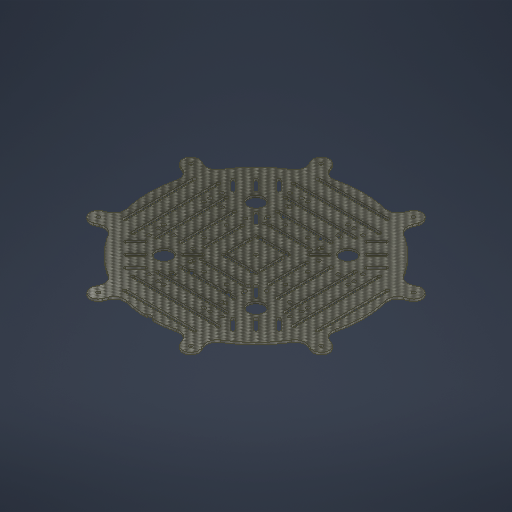
# Autodesk Inventor part: Body_Center_Plate
Saved by Autodesk Inventor 2025 (Build 290162010, 162A)
## iProperties
Created: 2023-12-04
Part Number: Body_Center_Plate
Material: GFRC
Document SubType Name: Modeling
Designer: dzw04
Density: 1.7 g/cm^3
Appearance: Carbon Fiber 1
Mass: 94.6856 g
Surface Area: 657.949 cm^2
Volume: 55.6974 cm^3
Author: dzw04
Autodesk Inventor part; units mm, degrees
ref_plane "YZ Plane" through (0, 0, 0) normal (1, 0, 0) x (0, 1, 0)
ref_plane "XZ Plane" through (0, 0, 0) normal (0, 1, 0) x (-1, 0, 0)
ref_plane "XY Plane" through (0, 0, 0) normal (0, 0, 1) x (1, 0, 0)
sketch "Sketch1" plane through (0, 0, 0) normal (0, 1, 0) x (-1, 0, 0)
  circle A0 centre (165, 165) radius 1.6
  circle A1 centre (121.9481, 268.9364) radius 1.6
  circle A2 centre (61.0636, 208.0519) radius 1.6
  circle A3 centre (61.0636, 121.9481) radius 1.6
  circle A4 centre (121.9481, 61.0636) radius 1.6
  circle A5 centre (208.0519, 61.0636) radius 1.6
  circle A6 centre (268.9364, 121.9481) radius 1.6
  circle A7 centre (268.9364, 208.0519) radius 1.6
  circle A8 centre (208.0519, 268.9364) radius 1.6
  arc A9 (160.6158, 264.9038) -> (141.9171, 262.2994) centre (165, 165) ccw
  arc A10 (130.37, 268.2025) -> (141.9171, 262.2994) centre (139.6088, 272.0294) ccw
  line L0 (130.37, 268.2025) -> (128.8772, 271.8066)
  arc A11 (128.8772, 271.8066) -> (115.019, 266.0663) centre (121.9481, 268.9364) ccw
  line L1 (115.019, 266.0663) -> (116.5119, 262.4623)
  arc A12 (112.521, 250.1231) -> (116.5119, 262.4623) centre (107.2731, 258.6355) ccw
  arc A13 (112.521, 250.1231) -> (79.8769, 217.479) centre (165, 165) ccw
  arc A14 (67.5377, 213.4881) -> (79.8769, 217.479) centre (71.3645, 222.7269) ccw
  line L2 (67.5377, 213.4881) -> (63.9337, 214.981)
  arc A15 (63.9337, 214.981) -> (58.1934, 201.1228) centre (61.0636, 208.0519) ccw
  line L3 (58.1934, 201.1228) -> (61.7975, 199.63)
  arc A16 (67.7006, 188.0829) -> (61.7975, 199.63) centre (57.9706, 190.3912) ccw
  arc A17 (67.7006, 188.0829) -> (67.7006, 141.9171) centre (165, 165) ccw
  arc A18 (61.7975, 130.37) -> (67.7006, 141.9171) centre (57.9706, 139.6088) ccw
  line L4 (61.7975, 130.37) -> (58.1934, 128.8772)
  arc A19 (58.1934, 128.8772) -> (63.9337, 115.019) centre (61.0636, 121.9481) ccw
  line L5 (63.9337, 115.019) -> (67.5377, 116.5119)
  arc A20 (79.8769, 112.521) -> (67.5377, 116.5119) centre (71.3645, 107.2731) ccw
  arc A21 (79.8769, 112.521) -> (112.521, 79.8769) centre (165, 165) ccw
  arc A22 (116.5119, 67.5377) -> (112.521, 79.8769) centre (107.2731, 71.3645) ccw
  line L6 (116.5119, 67.5377) -> (115.019, 63.9337)
  arc A23 (115.019, 63.9337) -> (128.8772, 58.1934) centre (121.9481, 61.0636) ccw
  line L7 (128.8772, 58.1934) -> (130.37, 61.7975)
  arc A24 (141.9171, 67.7006) -> (130.37, 61.7975) centre (139.6088, 57.9706) ccw
  arc A25 (141.9171, 67.7006) -> (188.0829, 67.7006) centre (165, 165) ccw
  arc A26 (199.63, 61.7975) -> (188.0829, 67.7006) centre (190.3912, 57.9706) ccw
  line L8 (199.63, 61.7975) -> (201.1228, 58.1934)
  arc A27 (201.1228, 58.1934) -> (214.981, 63.9337) centre (208.0519, 61.0636) ccw
  line L9 (214.981, 63.9337) -> (213.4881, 67.5377)
  arc A28 (217.479, 79.8769) -> (213.4881, 67.5377) centre (222.7269, 71.3645) ccw
  arc A29 (217.479, 79.8769) -> (250.1231, 112.521) centre (165, 165) ccw
  arc A30 (262.4623, 116.5119) -> (250.1231, 112.521) centre (258.6355, 107.2731) ccw
  line L10 (262.4623, 116.5119) -> (266.0663, 115.019)
  arc A31 (266.0663, 115.019) -> (271.8066, 128.8772) centre (268.9364, 121.9481) ccw
  line L11 (271.8066, 128.8772) -> (268.2025, 130.37)
  arc A32 (262.2994, 141.9171) -> (268.2025, 130.37) centre (272.0294, 139.6088) ccw
  arc A33 (262.2994, 141.9171) -> (262.2994, 188.0829) centre (165, 165) ccw
  arc A34 (268.2025, 199.63) -> (262.2994, 188.0829) centre (272.0294, 190.3912) ccw
  line L12 (268.2025, 199.63) -> (271.8066, 201.1228)
  arc A35 (271.8066, 201.1228) -> (266.0663, 214.981) centre (268.9364, 208.0519) ccw
  line L13 (266.0663, 214.981) -> (262.4623, 213.4881)
  arc A36 (250.1231, 217.479) -> (262.4623, 213.4881) centre (258.6355, 222.7269) ccw
  arc A37 (250.1231, 217.479) -> (217.479, 250.1231) centre (165, 165) ccw
  arc A38 (213.4881, 262.4623) -> (217.479, 250.1231) centre (222.7269, 258.6355) ccw
  line L14 (213.4881, 262.4623) -> (214.981, 266.0663)
  arc A39 (214.981, 266.0663) -> (201.1228, 271.8066) centre (208.0519, 268.9364) ccw
  line L15 (201.1228, 271.8066) -> (199.63, 268.2025)
  arc A40 (188.0829, 262.2994) -> (199.63, 268.2025) centre (190.3912, 272.0294) ccw
  arc A41 (188.0829, 262.2994) -> (169.3842, 264.9038) centre (165, 165) ccw
  arc A42 (169.3842, 264.9038) -> (167.1373, 263.7031) centre (169.2746, 262.4062) ccw
  arc A43 (162.8627, 263.7031) -> (167.1373, 263.7031) centre (165, 265) ccw
  arc A44 (162.8627, 263.7031) -> (160.6158, 264.9038) centre (160.7254, 262.4062) ccw
  circle A45 centre (207.8601, 207.8601) radius 7.5
  arc A46 (215.6383, 217.7596) -> (217.7596, 215.6383) centre (216.6989, 216.6989) ccw
  line L16 (215.6383, 217.7596) -> (224.5498, 226.6711)
  arc A47 (226.6711, 224.5498) -> (224.5498, 226.6711) centre (225.6104, 225.6104) ccw
  line L17 (226.6711, 224.5498) -> (217.7596, 215.6383)
  arc A48 (189.0491, 191.1704) -> (191.1704, 189.0491) centre (190.1098, 190.1098) ccw
  line L18 (189.0491, 191.1704) -> (197.9606, 200.0819)
  arc A49 (200.0819, 197.9606) -> (197.9606, 200.0819) centre (199.0213, 199.0213) ccw
  line L19 (200.0819, 197.9606) -> (191.1704, 189.0491)
  circle A50 centre (122.1399, 207.8601) radius 7.5
  arc A51 (112.2404, 215.6383) -> (114.3617, 217.7596) centre (113.3011, 216.6989) ccw
  line L20 (112.2404, 215.6383) -> (103.3289, 224.5498)
  arc A52 (105.4502, 226.6711) -> (103.3289, 224.5498) centre (104.3896, 225.6104) ccw
  line L21 (105.4502, 226.6711) -> (114.3617, 217.7596)
  arc A53 (138.8296, 189.0491) -> (140.9509, 191.1704) centre (139.8902, 190.1098) ccw
  line L22 (138.8296, 189.0491) -> (129.9181, 197.9606)
  arc A54 (132.0394, 200.0819) -> (129.9181, 197.9606) centre (130.9787, 199.0213) ccw
  line L23 (132.0394, 200.0819) -> (140.9509, 191.1704)
  circle A55 centre (122.1399, 122.1399) radius 7.5
  arc A56 (114.3617, 112.2404) -> (112.2404, 114.3617) centre (113.3011, 113.3011) ccw
  line L24 (114.3617, 112.2404) -> (105.4502, 103.3289)
  arc A57 (103.3289, 105.4502) -> (105.4502, 103.3289) centre (104.3896, 104.3896) ccw
  line L25 (103.3289, 105.4502) -> (112.2404, 114.3617)
  arc A58 (140.9509, 138.8296) -> (138.8296, 140.9509) centre (139.8902, 139.8902) ccw
  line L26 (140.9509, 138.8296) -> (132.0394, 129.9181)
  arc A59 (129.9181, 132.0394) -> (132.0394, 129.9181) centre (130.9787, 130.9787) ccw
  line L27 (129.9181, 132.0394) -> (138.8296, 140.9509)
  circle A60 centre (207.8601, 122.1399) radius 7.5
  arc A61 (217.7596, 114.3617) -> (215.6383, 112.2404) centre (216.6989, 113.3011) ccw
  line L28 (217.7596, 114.3617) -> (226.6711, 105.4502)
  arc A62 (224.5498, 103.3289) -> (226.6711, 105.4502) centre (225.6104, 104.3896) ccw
  line L29 (224.5498, 103.3289) -> (215.6383, 112.2404)
  arc A63 (191.1704, 140.9509) -> (189.0491, 138.8296) centre (190.1098, 139.8902) ccw
  line L30 (191.1704, 140.9509) -> (200.0819, 132.0394)
  arc A64 (197.9606, 129.9181) -> (200.0819, 132.0394) centre (199.0213, 130.9787) ccw
  line L31 (197.9606, 129.9181) -> (189.0491, 138.8296)
  arc A65 (207.153, 103.7551) -> (205.0317, 101.6338) centre (206.0923, 102.6945) ccw
  line L32 (207.153, 103.7551) -> (216.0645, 94.8436)
  arc A66 (213.9432, 92.7223) -> (216.0645, 94.8436) centre (215.0038, 93.783) ccw
  line L33 (213.9432, 92.7223) -> (205.0317, 101.6338)
  line L34 (237.2777, 116.0568) -> (228.3662, 124.9683)
  arc A67 (228.3662, 124.9683) -> (226.2449, 122.847) centre (227.3055, 123.9077) ccw
  line L35 (226.2449, 122.847) -> (235.1564, 113.9355)
  arc A68 (235.1564, 113.9355) -> (237.2777, 116.0568) centre (236.217, 114.9962) ccw
  arc A69 (103.7551, 122.847) -> (101.6338, 124.9683) centre (102.6945, 123.9077) ccw
  line L36 (103.7551, 122.847) -> (94.8436, 113.9355)
  arc A70 (92.7223, 116.0568) -> (94.8436, 113.9355) centre (93.783, 114.9962) ccw
  line L37 (92.7223, 116.0568) -> (101.6338, 124.9683)
  line L38 (116.0568, 92.7223) -> (124.9683, 101.6338)
  arc A71 (124.9683, 101.6338) -> (122.847, 103.7551) centre (123.9077, 102.6945) ccw
  line L39 (122.847, 103.7551) -> (113.9355, 94.8436)
  arc A72 (113.9355, 94.8436) -> (116.0568, 92.7223) centre (114.9962, 93.783) ccw
  arc A73 (122.847, 226.2449) -> (124.9683, 228.3662) centre (123.9077, 227.3055) ccw
  line L40 (122.847, 226.2449) -> (113.9355, 235.1564)
  arc A74 (116.0568, 237.2777) -> (113.9355, 235.1564) centre (114.9962, 236.217) ccw
  line L41 (116.0568, 237.2777) -> (124.9683, 228.3662)
  line L42 (103.7551, 207.153) -> (94.8436, 216.0645)
  arc A75 (94.8436, 216.0645) -> (92.7223, 213.9432) centre (93.783, 215.0038) ccw
  line L43 (92.7223, 213.9432) -> (101.6338, 205.0317)
  arc A76 (101.6338, 205.0317) -> (103.7551, 207.153) centre (102.6945, 206.0923) ccw
  arc A77 (226.2449, 207.153) -> (228.3662, 205.0317) centre (227.3055, 206.0923) ccw
  line L44 (226.2449, 207.153) -> (235.1564, 216.0645)
  arc A78 (237.2777, 213.9432) -> (235.1564, 216.0645) centre (236.217, 215.0038) ccw
  line L45 (237.2777, 213.9432) -> (228.3662, 205.0317)
  line L46 (213.9432, 237.2777) -> (205.0317, 228.3662)
  arc A79 (205.0317, 228.3662) -> (207.153, 226.2449) centre (206.0923, 227.3055) ccw
  line L47 (207.153, 226.2449) -> (216.0645, 235.1564)
  arc A80 (216.0645, 235.1564) -> (213.9432, 237.2777) centre (215.0038, 236.217) ccw
  arc A81 (197.5, 73.5) -> (197.5, 76.5) centre (197.5, 75) ccw
  line L48 (197.5, 73.5) -> (132.5, 73.5)
  arc A82 (132.5, 76.5) -> (132.5, 73.5) centre (132.5, 75) ccw
  line L49 (132.5, 76.5) -> (197.5, 76.5)
  line L50 (73.5, 197.5) -> (73.5, 132.5)
  arc A83 (73.5, 132.5) -> (76.5, 132.5) centre (75, 132.5) ccw
  line L51 (76.5, 132.5) -> (76.5, 197.5)
  arc A84 (76.5, 197.5) -> (73.5, 197.5) centre (75, 197.5) ccw
  line L52 (256.5, 197.5) -> (256.5, 132.5)
  arc A85 (253.5, 132.5) -> (256.5, 132.5) centre (255, 132.5) ccw
  line L53 (253.5, 132.5) -> (253.5, 197.5)
  arc A86 (256.5, 197.5) -> (253.5, 197.5) centre (255, 197.5) ccw
  line L54 (132.5, 253.5) -> (197.5, 253.5)
  arc A87 (197.5, 253.5) -> (197.5, 256.5) centre (197.5, 255) ccw
  line L55 (197.5, 256.5) -> (132.5, 256.5)
  arc A88 (132.5, 256.5) -> (132.5, 253.5) centre (132.5, 255) ccw
  line L56 (132.5, 223.5) -> (197.5, 223.5)
  arc A89 (197.5, 223.5) -> (197.5, 226.5) centre (197.5, 225) ccw
  line L57 (197.5, 226.5) -> (132.5, 226.5)
  arc A90 (132.5, 226.5) -> (132.5, 223.5) centre (132.5, 225) ccw
  line L58 (182.5, 196.5) -> (147.5, 196.5)
  arc A91 (147.5, 196.5) -> (147.5, 193.5) centre (147.5, 195) ccw
  line L59 (147.5, 193.5) -> (182.5, 193.5)
  arc A92 (182.5, 193.5) -> (182.5, 196.5) centre (182.5, 195) ccw
  line L60 (205, 241.5) -> (125, 241.5)
  arc A93 (125, 241.5) -> (125, 238.5) centre (125, 240) ccw
  line L61 (125, 238.5) -> (205, 238.5)
  arc A94 (205, 238.5) -> (205, 241.5) centre (205, 240) ccw
  arc A95 (197.5, 103.5) -> (197.5, 106.5) centre (197.5, 105) ccw
  line L62 (197.5, 103.5) -> (132.5, 103.5)
  arc A96 (132.5, 106.5) -> (132.5, 103.5) centre (132.5, 105) ccw
  line L63 (132.5, 106.5) -> (197.5, 106.5)
  arc A97 (182.5, 133.5) -> (182.5, 136.5) centre (182.5, 135) ccw
  line L64 (182.5, 133.5) -> (147.5, 133.5)
  arc A98 (147.5, 136.5) -> (147.5, 133.5) centre (147.5, 135) ccw
  line L65 (147.5, 136.5) -> (182.5, 136.5)
  arc A99 (205, 88.5) -> (205, 91.5) centre (205, 90) ccw
  line L66 (205, 88.5) -> (125, 88.5)
  arc A100 (125, 91.5) -> (125, 88.5) centre (125, 90) ccw
  line L67 (125, 91.5) -> (205, 91.5)
  line L68 (103.5, 197.5) -> (103.5, 132.5)
  arc A101 (103.5, 132.5) -> (106.5, 132.5) centre (105, 132.5) ccw
  line L69 (106.5, 132.5) -> (106.5, 197.5)
  arc A102 (106.5, 197.5) -> (103.5, 197.5) centre (105, 197.5) ccw
  line L70 (133.5, 182.5) -> (133.5, 147.5)
  arc A103 (133.5, 147.5) -> (136.5, 147.5) centre (135, 147.5) ccw
  line L71 (136.5, 147.5) -> (136.5, 182.5)
  arc A104 (136.5, 182.5) -> (133.5, 182.5) centre (135, 182.5) ccw
  line L72 (118.5, 190) -> (118.5, 140)
  arc A105 (118.5, 140) -> (121.5, 140) centre (120, 140) ccw
  line L73 (121.5, 140) -> (121.5, 190)
  arc A106 (121.5, 190) -> (118.5, 190) centre (120, 190) ccw
  line L74 (91.5, 125) -> (91.5, 205)
  arc A107 (91.5, 205) -> (88.5, 205) centre (90, 205) ccw
  line L75 (88.5, 205) -> (88.5, 125)
  arc A108 (88.5, 125) -> (91.5, 125) centre (90, 125) ccw
  line L76 (151.5, 155) -> (151.5, 175)
  arc A109 (151.5, 175) -> (148.5, 175) centre (150, 175) ccw
  line L77 (148.5, 175) -> (148.5, 155)
  arc A110 (148.5, 155) -> (151.5, 155) centre (150, 155) ccw
  line L78 (226.5, 197.5) -> (226.5, 132.5)
  arc A111 (223.5, 132.5) -> (226.5, 132.5) centre (225, 132.5) ccw
  line L79 (223.5, 132.5) -> (223.5, 197.5)
  arc A112 (226.5, 197.5) -> (223.5, 197.5) centre (225, 197.5) ccw
  arc A113 (196.5, 182.5) -> (193.5, 182.5) centre (195, 182.5) ccw
  line L80 (196.5, 182.5) -> (196.5, 147.5)
  arc A114 (193.5, 147.5) -> (196.5, 147.5) centre (195, 147.5) ccw
  line L81 (193.5, 147.5) -> (193.5, 182.5)
  arc A115 (211.5, 190) -> (208.5, 190) centre (210, 190) ccw
  line L82 (211.5, 190) -> (211.5, 140)
  arc A116 (208.5, 140) -> (211.5, 140) centre (210, 140) ccw
  line L83 (208.5, 140) -> (208.5, 190)
  line L84 (238.5, 125) -> (238.5, 205)
  arc A117 (241.5, 205) -> (238.5, 205) centre (240, 205) ccw
  line L85 (241.5, 205) -> (241.5, 125)
  arc A118 (238.5, 125) -> (241.5, 125) centre (240, 125) ccw
  line L86 (181.5, 175) -> (181.5, 155)
  arc A119 (178.5, 155) -> (181.5, 155) centre (180, 155) ccw
  line L87 (178.5, 155) -> (178.5, 175)
  arc A120 (181.5, 175) -> (178.5, 175) centre (180, 175) ccw
  arc A121 (151.5434, 148.3095) -> (154.0566, 148.3095) centre (152.8, 149.3) ccw
  arc A122 (151.5434, 148.3095) -> (151.1508, 148.5) centre (151.1508, 148) ccw
  line L88 (151.1508, 148.5) -> (150, 148.5)
  arc A123 (150, 151.5) -> (150, 148.5) centre (150, 150) ccw
  line L89 (150, 151.5) -> (180, 151.5)
  arc A124 (180, 148.5) -> (180, 151.5) centre (180, 150) ccw
  line L90 (180, 148.5) -> (178.8492, 148.5)
  arc A125 (178.8492, 148.5) -> (178.4566, 148.3095) centre (178.8492, 148) ccw
  arc A126 (175.9434, 148.3095) -> (178.4566, 148.3095) centre (177.2, 149.3) ccw
  arc A127 (175.9434, 148.3095) -> (175.5508, 148.5) centre (175.5508, 148) ccw
  line L91 (175.5508, 148.5) -> (154.4492, 148.5)
  arc A128 (154.4492, 148.5) -> (154.0566, 148.3095) centre (154.4492, 148) ccw
  line L92 (175.5508, 181.5) -> (154.4492, 181.5)
  arc A129 (154.0566, 181.6905) -> (154.4492, 181.5) centre (154.4492, 182) ccw
  arc A130 (154.0566, 181.6905) -> (151.5434, 181.6905) centre (152.8, 180.7) ccw
  arc A131 (151.1508, 181.5) -> (151.5434, 181.6905) centre (151.1508, 182) ccw
  line L93 (151.1508, 181.5) -> (150, 181.5)
  arc A132 (150, 181.5) -> (150, 178.5) centre (150, 180) ccw
  line L94 (150, 178.5) -> (180, 178.5)
  arc A133 (180, 178.5) -> (180, 181.5) centre (180, 180) ccw
  line L95 (180, 181.5) -> (178.8492, 181.5)
  arc A134 (178.4566, 181.6905) -> (178.8492, 181.5) centre (178.8492, 182) ccw
  arc A135 (178.4566, 181.6905) -> (175.9434, 181.6905) centre (177.2, 180.7) ccw
  arc A136 (175.5508, 181.5) -> (175.9434, 181.6905) centre (175.5508, 182) ccw
  line L96 (180.6, 122.5) -> (180.6, 122)
  arc A137 (180.1, 121.5) -> (180.6, 122) centre (180.1, 122) ccw
  line L97 (180.1, 121.5) -> (149.9, 121.5)
  arc A138 (149.4, 122) -> (149.9, 121.5) centre (149.9, 122) ccw
  line L98 (149.4, 122) -> (149.4, 122.5)
  arc A139 (149.4, 122.5) -> (146.2, 122.5) centre (147.8, 122.5) ccw
  line L99 (146.2, 122.5) -> (146.2, 122)
  arc A140 (145.7, 121.5) -> (146.2, 122) centre (145.7, 122) ccw
  line L100 (145.7, 121.5) -> (140, 121.5)
  arc A141 (140, 121.5) -> (140, 118.5) centre (140, 120) ccw
  line L101 (140, 118.5) -> (190, 118.5)
  arc A142 (190, 118.5) -> (190, 121.5) centre (190, 120) ccw
  line L102 (190, 121.5) -> (184.3, 121.5)
  arc A143 (183.8, 122) -> (184.3, 121.5) centre (184.3, 122) ccw
  line L103 (183.8, 122) -> (183.8, 122.5)
  arc A144 (183.8, 122.5) -> (180.6, 122.5) centre (182.2, 122.5) ccw
  line L104 (149.4, 207.5) -> (149.4, 208)
  arc A145 (149.9, 208.5) -> (149.4, 208) centre (149.9, 208) ccw
  line L105 (149.9, 208.5) -> (180.1, 208.5)
  arc A146 (180.6, 208) -> (180.1, 208.5) centre (180.1, 208) ccw
  line L106 (180.6, 208) -> (180.6, 207.5)
  arc A147 (180.6, 207.5) -> (183.754, 207.881) centre (182.2, 207.5) ccw
  arc A148 (184.2396, 208.5) -> (183.754, 207.881) centre (184.2396, 208) ccw
  line L107 (184.2396, 208.5) -> (190, 208.5)
  arc A149 (190, 208.5) -> (190, 211.5) centre (190, 210) ccw
  line L108 (190, 211.5) -> (140, 211.5)
  arc A150 (140, 211.5) -> (140, 208.5) centre (140, 210) ccw
  line L109 (140, 208.5) -> (145.7, 208.5)
  arc A151 (146.2, 208) -> (145.7, 208.5) centre (145.7, 208) ccw
  line L110 (146.2, 208) -> (146.2, 207.5)
  arc A152 (146.2, 207.5) -> (149.4, 207.5) centre (147.8, 207.5) ccw
  circle A153 centre (189.375, 232.125) radius 1.6
  circle A154 centre (140.625, 232.125) radius 1.6
  circle A155 centre (97.875, 140.625) radius 1.6
  circle A156 centre (97.875, 189.375) radius 1.6
  circle A157 centre (189.375, 97.875) radius 1.6
  circle A158 centre (140.625, 97.875) radius 1.6
  circle A159 centre (232.125, 140.625) radius 1.6
  circle A160 centre (232.125, 189.375) radius 1.6
  circle A161 centre (219, 142.5) radius 1.6
  circle A162 centre (111, 142.5) radius 1.6
  circle A163 centre (219, 187.5) radius 1.6
  circle A164 centre (111, 187.5) radius 1.6
  circle A165 centre (98.0016, 183.7383) radius 1.6
  circle A166 centre (146.2617, 231.9984) radius 1.6
  circle A167 centre (199.125, 189.375) radius 1.6
  circle A168 centre (130.875, 189.375) radius 1.6
  circle A169 centre (130.875, 230.625) radius 1.6
  circle A170 centre (199.125, 230.625) radius 1.6
  circle A171 centre (127.1698, 175.4298) radius 1.6
  circle A172 centre (175.4298, 127.1698) radius 1.6
  circle A173 centre (127.1698, 154.5702) radius 1.6
  circle A174 centre (202.8302, 175.4298) radius 1.6
  circle A175 centre (183.7383, 98.0016) radius 1.6
  circle A176 centre (130.875, 140.625) radius 1.6
  circle A177 centre (199.125, 140.625) radius 1.6
  circle A178 centre (199.125, 99.375) radius 1.6
  circle A179 centre (130.875, 99.375) radius 1.6
  circle A180 centre (202.8302, 154.5702) radius 1.6
  circle A181 centre (154.5702, 202.8302) radius 1.6
  circle A182 centre (146.2617, 98.0016) radius 1.6
  circle A183 centre (98.0016, 146.2617) radius 1.6
  circle A184 centre (99.375, 130.875) radius 1.6
  circle A185 centre (99.375, 199.125) radius 1.6
  circle A186 centre (183.7383, 231.9984) radius 1.6
  circle A187 centre (231.9984, 183.7383) radius 1.6
  circle A188 centre (230.625, 199.125) radius 1.6
  circle A189 centre (230.625, 130.875) radius 1.6
  circle A190 centre (175.4298, 202.8302) radius 1.6
  circle A191 centre (231.9984, 146.2617) radius 1.6
  circle A192 centre (154.5702, 127.1698) radius 1.6
  arc A193 (187.1862, 112.5689) -> (187.8138, 109.4311) centre (187.5, 111) ccw
  line L111 (187.1862, 112.5689) -> (189.6862, 113.0689)
  arc A194 (190.3138, 109.9311) -> (189.6862, 113.0689) centre (190, 111.5) ccw
  line L112 (190.3138, 109.9311) -> (187.8138, 109.4311)
  line L113 (142.8138, 112.5689) -> (140.3138, 113.0689)
  arc A195 (140.3138, 113.0689) -> (139.6862, 109.9311) centre (140, 111.5) ccw
  line L114 (139.6862, 109.9311) -> (142.1862, 109.4311)
  arc A196 (142.1862, 109.4311) -> (142.8138, 112.5689) centre (142.5, 111) ccw
  circle A197 centre (186.5, 194) radius 1.6
  circle A198 centre (143.5, 194) radius 1.6
  circle A199 centre (143.5, 136) radius 1.6
  circle A200 centre (186.5, 136) radius 1.6
  line L115 (187.8277, 130.4678) -> (188.4527, 128.0928)
  arc A201 (190.9223, 131.2822) -> (187.8277, 130.4678) centre (189.375, 130.875) ccw
  arc A202 (188.4527, 128.0928) -> (191.5473, 128.9072) centre (190, 128.5) ccw
  line L116 (139.0777, 131.2822) -> (138.4527, 128.9072)
  arc A203 (138.4527, 128.9072) -> (141.5473, 128.0928) centre (140, 128.5) ccw
  line L117 (141.5473, 128.0928) -> (142.1723, 130.4678)
  arc A204 (142.1723, 130.4678) -> (139.0777, 131.2822) centre (140.625, 130.875) ccw
  line L118 (191.5473, 128.9072) -> (190.9223, 131.2822)
  arc A205 (142.8138, 217.4311) -> (142.1862, 220.5689) centre (142.5, 219) ccw
  line L119 (142.8138, 217.4311) -> (140.3138, 216.9311)
  arc A206 (139.6862, 220.0689) -> (140.3138, 216.9311) centre (140, 218.5) ccw
  line L120 (139.6862, 220.0689) -> (142.1862, 220.5689)
  line L121 (187.1862, 217.4311) -> (189.6862, 216.9311)
  arc A207 (189.6862, 216.9311) -> (190.3138, 220.0689) centre (190, 218.5) ccw
  line L122 (190.3138, 220.0689) -> (187.8138, 220.5689)
  arc A208 (187.8138, 220.5689) -> (187.1862, 217.4311) centre (187.5, 219) ccw
  line L123 (190.9223, 198.7178) -> (191.5473, 201.0928)
  arc A209 (191.5473, 201.0928) -> (188.4527, 201.9072) centre (190, 201.5) ccw
  line L124 (188.4527, 201.9072) -> (187.8277, 199.5322)
  arc A210 (187.8277, 199.5322) -> (190.9223, 198.7178) centre (189.375, 199.125) ccw
  arc A211 (139.0777, 198.7178) -> (142.1723, 199.5322) centre (140.625, 199.125) ccw
  line L125 (139.0777, 198.7178) -> (138.4527, 201.0928)
  arc A212 (141.5473, 201.9072) -> (138.4527, 201.0928) centre (140, 201.5) ccw
  line L126 (141.5473, 201.9072) -> (142.1723, 199.5322)
  point P0 (0, 0)
  point P1 (141.9171, 262.2994)
  point P2 (115.019, 266.0663)
  point P3 (79.8769, 217.479)
  point P4 (67.5377, 213.4881)
  point P5 (67.7006, 141.9171)
  point P6 (63.9337, 115.019)
  point P7 (112.521, 79.8769)
  point P8 (188.0829, 67.7006)
  point P9 (214.981, 63.9337)
  point P10 (250.1231, 112.521)
  point P11 (271.8066, 128.8772)
  point P12 (266.0663, 214.981)
  point P13 (217.479, 250.1231)
  point P14 (201.1228, 271.8066)
  point P15 (169.3842, 264.9038)
  point P16 (142.1723, 199.5322)
  point P17 (188.4527, 201.9072)
  point P18 (191.5473, 128.9072)
  point P19 (140, 208.5)
  point P20 (190, 211.5)
  point P21 (190, 121.5)
  point P22 (140, 118.5)
  point P23 (145.7, 121.5)
  point P24 (146.2, 122.5)
  point P25 (180, 181.5)
  point P26 (150, 178.5)
  point P27 (175.9434, 181.6905)
  point P28 (151.5434, 148.3095)
  point P29 (208.5, 190)
  point P30 (211.5, 190)
  point P31 (193.5, 147.5)
  point P32 (193.5, 182.5)
  point P33 (196.5, 182.5)
  point P34 (223.5, 132.5)
  point P35 (148.5, 175)
  point P36 (121.5, 140)
  point P37 (106.5, 132.5)
  point P38 (125, 91.5)
  point P39 (205, 91.5)
  point P40 (182.5, 136.5)
  point P41 (125, 238.5)
  point P42 (197.5, 226.5)
  point P43 (197.5, 256.5)
  point P44 (253.5, 132.5)
  point P45 (76.5, 132.5)
  point P46 (132.5, 76.5)
  point P47 (207.153, 226.2449)
  point P48 (92.7223, 213.9432)
  point P49 (124.9683, 228.3662)
  point P50 (122.847, 103.7551)
  point P51 (101.6338, 124.9683)
  point P52 (226.2449, 122.847)
  point P53 (213.9432, 92.7223)
  point P54 (205.0317, 101.6338)
  point P55 (207.153, 103.7551)
  point P56 (189.0491, 138.8296)
  point P57 (215.6383, 112.2404)
  point P58 (217.7596, 114.3617)
  point P59 (138.8296, 140.9509)
  point P60 (112.2404, 114.3617)
  point P61 (132.0394, 200.0819)
  point P62 (140.9509, 191.1704)
  point P63 (105.4502, 226.6711)
  point P64 (114.3617, 217.7596)
  point P65 (217.7596, 215.6383)
  constraints: 312 point on circle, 254 end point, 213 centre point
extrude "Extrusion1" add sketch "Sketch1" along normal blind 2
equation "\"d0\" = ThicknessBodyCenterPlate"
equation "\"MountToMotorCenter\" = 0"
equation "\"ArmPosition\" = 5deg"
equation "\"BatteryWidth\" = 62"
equation "\"BatteryHeight\" = 76"
equation "\"ThicknessBodyOuterPlate\" = 2"
equation "\"ThicknessBodyCenterPlate\" = 2"
equation "\"ThicknessLegLoadpipePlate\" = 2"
equation "\"ThicknessBatteryTray\" = 2"
equation "\"ThicknessBatteryTopTray\" = 1"
equation "\"LandingGearStabilityBar\" = 525"
equation "\"StartAngleArm\" = 45deg"
equation "\"MotorMountCenter\" = 71.5"
body "Solid1"
